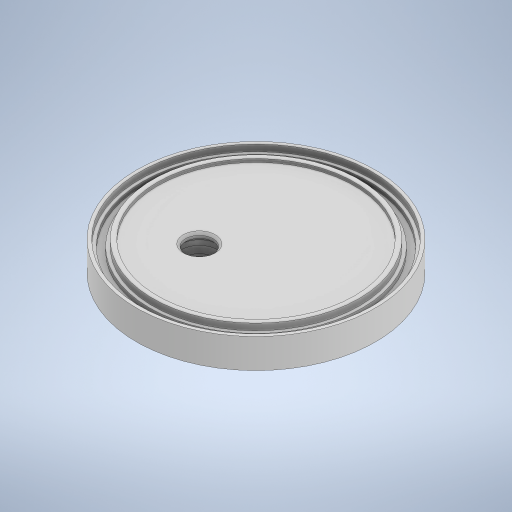
# Autodesk Inventor part: tubesheet_no_splitter
Saved by Autodesk Inventor 2023.5 (Build 275446000, 446)
## iProperties
Created: 2025-05-24
Part Number: tubesheet_no_splitter
Material: Generic
Document SubType Name: Modeling
Designer: ryanj
Density: 1 g/cm^3
Appearance: Default
Author: ryanj
Autodesk Inventor part; units mm, degrees
ref_plane "YZ Plane" through (0, 0, 0) normal (1, 0, 0) x (0, 1, 0)
ref_plane "XZ Plane" through (0, 0, 0) normal (0, 1, 0) x (-1, 0, 0)
ref_plane "XY Plane" through (0, 0, 0) normal (0, 0, 1) x (1, 0, 0)
sketch "Sketch1" plane through (0, 0, 0) normal (0, 1, 0) x (-1, 0, 0)
  circle A0 centre (0, 0) radius 36.5
  dimension "d0" = 73
  constraints: 1 centre point, 1 coincident
  measures "d0" diameter of A0
extrude "Extrusion1" add sketch "Sketch1" along normal blind 4.5
sketch "Sketch2" plane through (0, 4.5, 0) normal (0, 1, 0) x (1, 0, 0)
  circle A0 centre (0, 0) radius 35.5
  circle A1 centre (0, 0) radius 31.5
  dimension "d3" = 71
  dimension "d4" = 63
  constraints: 2 centre point, 2 coincident
  measures "d3" diameter of A0
  measures "d4" diameter of A1
extrude "Extrusion2" cut sketch "Sketch2" against normal blind 2
sketch "Sketch3" plane through (0, 2.5, 0) normal (0, 1, 0) x (1, 0, 0)
  circle A0 centre (0, 0) radius 34.5
  circle A1 centre (0, 0) radius 32.5
  dimension "d7" = 69
  dimension "d8" = 65
  constraints: 2 centre point, 2 coincident
  measures "d7" diameter of A0
  measures "d8" diameter of A1
extrude "Extrusion3" cut sketch "Sketch3" against normal blind 1.2
sketch "Sketch4" plane through (0, 4.5, 0) normal (0, 1, 0) x (1, 0, 0)
  circle A0 centre (0, 0) radius 30.085
  dimension "d11" = 60.17
  constraints: 1 centre point, 1 coincident
  measures "d11" diameter of A0
extrude "Extrusion4" cut sketch "Sketch4" against normal blind 1
sketch "Sketch5" plane through (0, 3.5, 0) normal (0, 1, 0) x (1, 0, 0)
  circle A0 centre (-8.3708, -8.9402) radius 4.2
  point P0 (0, 0)
  dimension "d14" = 8.4
  constraints: 1 centre point
  measures "d14" diameter of A0
extrude "Extrusion5" cut sketch "Sketch5" against normal blind 2.75
chamfer "Chamfer1" distance 0.69 angle 45 1 edges at (-12.5708, 3.5, 8.9402)
sketch "Sketch6" plane through (-8.3708, 0.75, 8.9402) normal (0, 1, 0) x (1, 0, 0)
  circle A0 centre (0, 0) radius 5.46
  point P0 (8.3708, 8.9402)
  dimension "d20" = 10.92
  constraints: 1 centre point
  measures "d20" diameter of A0
extrude "Extrusion6" cut sketch "Sketch6" against normal blind 0.75
chamfer "Chamfer2" distance 1.26 angle 45 1 edges at (-12.5708, 0.75, 8.9402)
mirror "Mirror3" about plane through (0, 0, 0) normal (0, 1, 0) of "Extrusion1", "Extrusion2", "Extrusion3", "Extrusion4", "Extrusion5", "Chamfer1", "Extrusion6", "Chamfer2"
body "Solid1"
